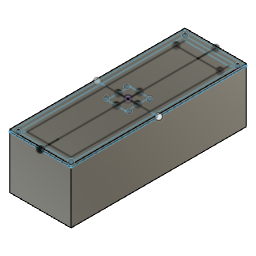
Pass_Cracker (Autodesk Fusion 360 design; units mm, degrees)
Autodesk Fusion 360 part; units mm, degrees
note: some values were not read from the file. Set by a fixed rule: the direction of a hole.
sketch "Sketch1" plane through (0, 0, 0) normal (0, 0, 1) x (1, 0, 0)
  line L0 (0, 0) -> (0, 80)
  line L1 (0, 0) -> (0, -80)
  line L2 (0, 0) -> (25, 0)
  line L3 (0, 0) -> (-25, 0)
  line L4 (-25, 0) -> (-35, 0)
  line L5 (25, 0) -> (35, 0)
  line L6 (0, 80) -> (0, 100)
  line L7 (0, -80) -> (0, -100)
  line L8 (0, 80) -> (0, 90)
  line L9 (0, -80) -> (0, -90)
  line L10 (0, 80) -> (25, 80)
  line L11 (0, 80) -> (-25, 80)
  line L12 (0, -90) -> (25, -90)
  line L13 (0, -90) -> (-25, -90)
  line L14 (-25, 90) -> (25, 90)
  line L15 (25, 90) -> (25, -90)
  line L16 (-25, -90) -> (-25, 90)
  line L17 (-35, 100) -> (35, 100)
  line L18 (35, 100) -> (35, -100)
  line L19 (35, -100) -> (-35, -100)
  line L20 (-35, -100) -> (-35, 100)
  line L21 (0, 0) -> (-11, 0)
  line L22 (0, 0) -> (11, 0)
  line L23 (0, 0) -> (0, 13.25)
  line L24 (0, 0) -> (0, -13.25)
  line L25 (-11, 13.25) -> (11, 13.25)
  line L26 (11, 13.25) -> (11, -13.25)
  line L27 (11, -13.25) -> (-11, -13.25)
  line L28 (-11, -13.25) -> (-11, 13.25)
  line L29 (-11, -13.25) -> (-13, -13.25)
  line L30 (-13, -13.25) -> (-13, -11.7)
  circle A0 centre (-13, -11.7) radius 1
  line L31 (-11, 13.25) -> (-13, 13.25)
  line L32 (-13, 13.25) -> (-13, 11.7)
  line L33 (11, 13.25) -> (13, 13.25)
  line L34 (13, 13.25) -> (13, 11.7)
  line L35 (11, -13.25) -> (13, -13.25)
  line L36 (13, -13.25) -> (13, -11.7)
  circle A1 centre (13, -11.7) radius 1
  circle A2 centre (13, 11.7) radius 1
  circle A3 centre (-13, 11.7) radius 1
  line L37 (25, 90) -> (35, 100)
  line L38 (25, -90) -> (35, -100)
  line L39 (-35, -100) -> (-25, -90)
  line L40 (-25, 90) -> (-35, 100)
  line L41 (-30, 95) -> (30, 95)
  line L42 (30, 95) -> (30, -95)
  line L43 (-30, -95) -> (30, -95)
  line L44 (-30, -95) -> (-30, 95)
  circle A4 centre (-30, 95) radius 1
  circle A5 centre (30, 95) radius 1
  circle A6 centre (-30, -95) radius 1
  circle A7 centre (30, -95) radius 1
  dimension "d70" = 80
  dimension "d71" = 80
  dimension "d73" = 25
  dimension "d74" = 25
  dimension "d75" = 10
  dimension "d77" = 10
  dimension "d79" = 20
  dimension "d80" = 20
  dimension "d81" = 25
  dimension "d82" = 25
  dimension "d83" = 25
  dimension "d84" = 25
  dimension "d89" = 11
  dimension "d90" = 11
  dimension "d91" = 13.25
  dimension "d92" = 13.25
  dimension "d93" = 2
  dimension "d94" = 1.55
  dimension "d95" = 2
  dimension "d96" = 2
  dimension "d98" = 1.55
  dimension "d99" = 2
  dimension "d100" = 1.55
  dimension "d101" = 2
  dimension "d102" = 1.55
  dimension "d103" = 2
  dimension "d104" = 2
  dimension "d105" = 2
  dimension "d112" = 2
  dimension "d113" = 2
  dimension "d114" = 2
  dimension "d115" = 2
  constraint coincident L0.start L1.start
  constraint vertical L0
  constraint parallel L0 L1
  constraint perpendicular L1 L2
  constraint perpendicular L0 L3
  constraint midpoint L6 L8.end
  constraint midpoint L7 L9.end
  constraint perpendicular L8 L10
  constraint perpendicular L8 L11
  constraint perpendicular L7 L12
  constraint perpendicular L7 L13
  constraint horizontal L14
  constraint vertical L15
  constraint vertical L16
  constraint horizontal L17
  constraint vertical L18
  constraint horizontal L19
  constraint vertical L20
  constraint perpendicular L0 L21
  constraint perpendicular L1 L22
  constraint perpendicular L2 L23
  constraint perpendicular L3 L24
  constraint horizontal L25
  constraint vertical L26
  constraint horizontal L27
  constraint vertical L28
  constraint perpendicular L28 L29
  constraint perpendicular L29 L30
  constraint coincident L30.end A0.centre
  constraint perpendicular L28 L31
  constraint perpendicular L31 L32
  constraint perpendicular L26 L33
  constraint perpendicular L33 L34
  constraint perpendicular L26 L35
  constraint perpendicular L35 L36
  constraint coincident L36.end A1.centre
  constraint coincident L34.end A2.centre
  constraint coincident L32.end A3.centre
  constraint perpendicular L38 L39
  constraint perpendicular L39 L40
  constraint midpoint L40 L41.start
  constraint midpoint L37 L41.end
  constraint perpendicular L6 L41
  constraint midpoint L38 L42.end
  constraint midpoint L39 L43.start
  constraint perpendicular L42 L43
  constraint coincident L41.start L44.end
  constraint coincident L41.end L42.start
  constraint coincident L43.start L44.start
  constraint coincident L42.end L43.end
  measures "d70" distance of L0.start L0.end
  measures "d71" distance of L0.start L1.end
  measures "d73" distance of L0.start L2.end
  measures "d74" distance of L0.start L3.end
  measures "d75" distance of L3.end L4.end
  measures "d77" distance of L2.end L5.end
  measures "d79" distance of L0.end L6.end
  measures "d80" distance of L1.end L7.end
  measures "d81" distance of L0.end L10.end
  measures "d82" distance of L0.end L11.end
  measures "d83" distance of L9.end L12.end
  measures "d84" distance of L9.end L13.end
  measures "d89" distance of L0.start L21.end
  measures "d90" distance of L0.start L22.end
  measures "d91" distance of L0.start L23.end
  measures "d92" distance of L0.start L24.end
  measures "d93" distance of L27.end L29.end
  measures "d94" distance of L29.end L30.end
  measures "d95" diameter of A0
  measures "d96" distance of L25.start L31.end
  measures "d98" distance of L31.end L32.end
  measures "d99" distance of L25.end L33.end
  measures "d100" distance of L33.end L34.end
  measures "d101" distance of L26.end L35.end
  measures "d102" distance of L35.end L36.end
  measures "d103" diameter of A1
  measures "d104" diameter of A2
  measures "d105" diameter of A3
  measures "d112" diameter of A4
  measures "d113" diameter of A5
  measures "d114" diameter of A6
  measures "d115" diameter of A7
extrude "Extrude7" add sketch "Sketch1" along normal blind 60 contours L5 L15 L37 L42 A5 | L5 L15 L38 L42 A7 | L4 L16 L39 L44 A6 | L4 L16 L40 L44 A4 | L6 L14 L40 L41 A4 | L6 L14 L37 L41 A5 | L7 L12 L38 L43 A7 | L7 L13 L39 L43 A6 | L5 L18 L37 L42 A5 | L5 L18 L38 L42 A7 | L4 L20 L39 L44 A6 | L4 L20 L40 L44 A4 | L6 L17 L40 L41 A4 | L6 L17 L37 L41 A5 | L7 L19 L38 L43 A7 | L7 L19 L39 L43 A6 | L37 L42 A5 | L37 L42 A5 | L38 L42 A7 | L38 L42 A7 | L38 L43 A7 | L39 L44 A6 | L39 L44 A6 | L40 L44 A4 | L40 L44 A4 | L39 L43 A6 | L40 L41 A4 | L40 L41 A4 | L37 L41 A5 | L37 L41 A5 | L39 L43 A6 | L38 L43 A7 makes body 1
extrude "Extrude8" add sketch "Sketch1" along normal blind 2 contours L0 L3 L21 L23 L25 L28 | L1 L2 L22 L24 L26 L27 | L0 L2 L22 L23 L25 L26 | L1 L3 L21 L24 L27 L28 | L0 L3 L11 L16 L25 L28 | L0 L2 L10 L15 L25 L26 | L1 L2 L7 L9 L12 L15 L26 L27 | L1 L3 L7 L9 L13 L16 L27 L28 | L6 L8 L11 L14 L16 | L6 L8 L10 L14 L15 | A0 | A1 | A2 | A3 bodies 1
extrude "Extrude9" cut sketch "Sketch1" along normal blind 10 contours L0 L3 L21 L23 L25 L28 | L1 L2 L22 L24 L26 L27 | L0 L2 L22 L23 L25 L26 | L1 L3 L21 L24 L27 L28 | L1 L2 L7 L9 L12 L15 L26 L27 | L5 L15 L38 L42 A7 | L7 L12 L38 L43 A7 | L5 L18 L38 L42 A7 | L7 L19 L38 L43 A7 | L38 L42 A7 | L38 L42 A7 | L38 L43 A7 | L38 L43 A7 | A0 | A1 | A2 | A3 bodies 1
extrude "Extrude10" add sketch "Sketch1" along normal blind 2 contours L1 L2 L7 L9 L12 L15 L26 L27 bodies 1
extrude "Extrude11" add sketch "Sketch1" along normal blind 10 contours L5 L15 L38 L42 A7 | L7 L12 L38 L43 A7 | L5 L18 L38 L42 A7 | L7 L19 L38 L43 A7 | L38 L42 A7 | L38 L42 A7 | L38 L43 A7 | L38 L43 A7 bodies 1
move_body "Move3" bodies 1 to x (1, 0, 0) y (0, 1, 0) z (0, 0, 1) at (0, 0, -60)
hole "Hole3" at (-30, -95, 0) at (30, -95, 0) at (-30, 95, 0) at (30, 95, 0) direction (0, 0, -1) diameter 1.623 depth 5 tip angle 118 bodies 1
thread "Thread2" "ISO Metric profile 2.0 M2x0.4 6H"
extrude "Extrude13" add sketch "Sketch1" along normal blind 2.5 separate body contours L0 L3 L21 L23 L25 L28 | L1 L2 L22 L24 L26 L27 | L0 L2 L22 L23 L25 L26 | L1 L3 L21 L24 L27 L28 | L0 L3 L11 L16 L25 L28 | L0 L2 L10 L15 L25 L26 | L1 L2 L7 L9 L12 L15 L26 L27 | L1 L3 L7 L9 L13 L16 L27 L28 | L6 L8 L11 L14 L16 | L6 L8 L10 L14 L15 | L5 L15 L37 L42 A5 | L5 L15 L38 L42 A7 | L4 L16 L39 L44 A6 | L4 L16 L40 L44 A4 | L6 L14 L40 L41 A4 | L6 L14 L37 L41 A5 | L7 L12 L38 L43 A7 | L7 L13 L39 L43 A6 | L5 L18 L37 L42 A5 | L5 L18 L38 L42 A7 | L4 L20 L39 L44 A6 | L4 L20 L40 L44 A4 | L6 L17 L40 L41 A4 | L6 L17 L37 L41 A5 | L7 L19 L38 L43 A7 | L7 L19 L39 L43 A6 | L37 L42 A5 | L37 L42 A5 | L38 L42 A7 | L38 L42 A7 | L38 L43 A7 | L39 L44 A6 | L39 L44 A6 | L40 L44 A4 | L40 L44 A4 | L39 L43 A6 | L40 L41 A4 | L40 L41 A4 | L37 L41 A5 | L37 L41 A5 | L39 L43 A6 | L38 L43 A7 | A0 | A1 | A2 | A3 makes body 2
hole "Hole4" at (-30, -95, 0) at (30, -95, 0) at (-30, 95, 0) at (30, 95, 0) direction (0, 0, 1) diameter 1.623 depth 22 tip angle 118 countersink diameter 4 countersink angle 90 bodies 2
equation "d134 = 9f75eacb-7ea7-4e95-b8bb-dd2b4acf215c"
